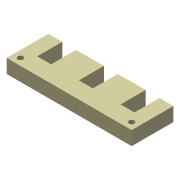
# Autodesk Inventor part: AgarMould
Saved by Autodesk Inventor 2013 (Build 170138000, 138)
## iProperties
Created: 2013-04-25
Part Number: AgarMould
Material: Nylon 6/6
Document SubType Name: Modeling
Designer: 120pa
Density: 1 g/cm^3
Author: 120pa
Autodesk Inventor part; units mm, degrees
ref_plane "YZ Plane" through (0, 0, 0) normal (1, 0, 0) x (0, 1, 0)
ref_plane "XZ Plane" through (0, 0, 0) normal (0, 1, 0) x (-1, 0, 0)
ref_plane "XY Plane" through (0, 0, 0) normal (0, 0, 1) x (1, 0, 0)
sketch "Sketch1" plane through (0, 0, 0) normal (0, 1, 0) x (-1, 0, 0)
  line L0 (-46.9942, 4.2491) -> (43.0058, 4.2491)
  line L1 (43.0058, 4.2491) -> (43.0058, -25.7509)
  line L2 (-46.9942, -25.7509) -> (-46.9942, 4.2491)
  line L3 (-26.9942, -25.7509) -> (-26.9942, -7.7509)
  line L4 (-26.9942, -7.7509) -> (-36.9942, -7.7509)
  line L5 (-36.9942, -7.7509) -> (-36.9942, -25.7509)
  line L6 (3.0058, -25.7509) -> (3.0058, -7.7509)
  line L7 (3.0058, -7.7509) -> (-6.9942, -7.7509)
  line L8 (-6.9942, -7.7509) -> (-6.9942, -25.7509)
  line L9 (33.0058, -25.7509) -> (33.0058, -7.7509)
  line L10 (33.0058, -7.7509) -> (23.0058, -7.7509)
  line L11 (23.0058, -7.7509) -> (23.0058, -25.7509)
  line L12 (-36.9942, -25.7509) -> (-46.9942, -25.7509)
  line L13 (-6.9942, -25.7509) -> (-26.9942, -25.7509)
  line L14 (43.0058, -25.7509) -> (33.0058, -25.7509)
  line L15 (23.0058, -25.7509) -> (3.0058, -25.7509)
  point P0 (0, 0)
  dimension "d0" = 90
  dimension "d3" = 30
  dimension "d4" = 10
  dimension "d5" = 20
  dimension "d6" = 20
  dimension "d7" = 18
  dimension "d8" = 18
  dimension "d9" = 18
  dimension "d10" = 18
  dimension "d11" = 18
  dimension "d12" = 10
  dimension "d13" = 10
  dimension "d14" = 10
  dimension "d17" = 18
  dimension "d18" = 30
  constraints: 32 end point, 8 parallel, 3 perpendicular, 1 horizontal
  measures "d0" distance of L0.start L0.end
  measures "d3" distance of L0.end L1.end
  measures "d4" distance between parallel lines of L2 L5
  measures "d5" distance between parallel lines of L8 L3
  measures "d6" distance between parallel lines of L11 L6
  measures "d7" distance of L4.end L5.end
  measures "d8" distance of L3.start L3.end
  measures "d9" distance of L7.end L8.end
  measures "d10" distance of L6.start L6.end
  measures "d11" distance of L10.end L11.end
  measures "d12" distance of L3.end L4.end
  measures "d13" distance of L6.end L7.end
  measures "d14" distance of L9.end L10.end
  measures "d17" distance of L9.start L9.end
  measures "d18" distance of L2.start L0.start
extrude "Extrusion1" add sketch "Sketch1" along normal blind 10
sketch "Sketch2" plane through (0, 10, 0) normal (0, 1, 0) x (1, 0, 0)
  line L0 (-43.0058, -4.2491) -> (46.9942, -4.2491) projected
  line L1 (46.9942, -4.2491) -> (46.9942, 25.7509) projected
  line L2 (-43.0058, 25.7509) -> (-43.0058, -4.2491) projected
  circle A0 centre (-38.0058, 0.7509) radius 2
  circle A1 centre (41.9942, 0.7509) radius 2
  point P0 (0, 0)
  dimension "d20" = 4
  dimension "d22" = 5
  dimension "d23" = 5
  dimension "d26" = 5
  dimension "d27" = 5
  dimension "d29" = 4
  constraints: 2 centre point
  measures "d20" diameter of A0
  measures "d22" distance from line of L0 A0.centre
  measures "d23" distance from line of L2 A0.centre
  measures "d26" distance from line of L0 A1.centre
  measures "d27" distance from line of A1.centre L1
  measures "d29" diameter of A1
extrude "Extrusion3" cut sketch "Sketch2" against normal blind 10
sketch "Sketch4" plane through (0, 0, 0) normal (0, -1, 0) x (1, 0, 0)
  line L0 (46.9942, 4.2491) -> (-43.0058, 4.2491) projected
  line L1 (-23.0058, -7.7509) -> (-23.0058, -25.7509) projected
  line L2 (26.9942, -25.7509) -> (26.9942, -7.7509) projected
  circle A0 centre (-13.0058, -10.7509) radius 2
  circle A1 centre (16.9942, -10.7509) radius 2
  point P0 (0, 0)
  dimension "d43" = 15
  dimension "d44" = 15
  dimension "d45" = 10
  dimension "d46" = 10
  dimension "d47" = 4
  dimension "d48" = 4
  constraints: 2 centre point
  measures "d43" distance from line of L0 A0.centre
  measures "d44" distance from line of A1.centre L0
  measures "d45" distance from line of A0.centre L1
  measures "d46" distance from line of A1.centre L2
  measures "d47" diameter of A0
  measures "d48" diameter of A1
extrude "Extrusion5" cut sketch "Sketch4" against normal blind 8
equation "\"d10\" = d7"
equation "\"d11\" = d7"
equation "\"d17\" = d7"
equation "\"d29\" = d20"
body "Solid1"
